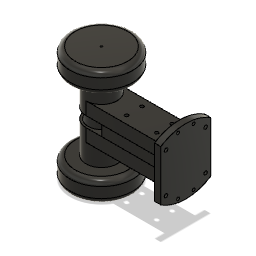
Supports projet fin de b3 (Autodesk Fusion 360 design; units mm, degrees)
Autodesk Fusion 360 part; units mm, degrees
note: some values were not read from the file. Set by a fixed rule: which sketch regions a step uses.
sketch "Esquisse1" plane through (0, 0, 0) normal (0, 1, 0) x (1, 0, 0)
  line L0 (0, 0) -> (0, 8.7) construction
  line L1 (0, -8.35) -> (1.45, -8.35)
  line L2 (0, 8.35) -> (1.45, 8.35)
  line L3 (0, -8.35) -> (-1.45, -8.35)
  circle A0 centre (0, 0) radius 2.9 construction
  circle A1 centre (0, 0) radius 9.45 construction
  line L4 (0, 0) -> (0, 1.3273)
  circle A2 centre (0, 0) radius 0.9
  line L5 (0, -8.7) -> (1.45, -8.7)
  line L6 (0, 8.35) -> (-1.45, 8.35)
  line L7 (0, 8.7) -> (-1.45, 8.7)
  line L8 (-6.6, 0) -> (-4.4, 0)
  circle A3 centre (5.5, 0.0034) radius 1.1
  line L9 (1.45, -8.7) -> (1.45, -8.35)
  line L10 (0, -8.7) -> (-1.45, -8.7)
  line L11 (1.45, 8.7) -> (1.45, 8.35)
  line L12 (-1.45, 8.7) -> (-1.45, 8.35)
  line L13 (0, 0) -> (-4.4, 0) construction
  circle A4 centre (-5.5, 0.0034) radius 1.1
  line L14 (0, 8.7) -> (1.45, 8.7)
  circle A5 centre (0, 0) radius 11.8 construction
  line L15 (0, 0) -> (0, 8.35) construction
  line L16 (-1.45, -8.7) -> (-1.45, -8.35)
  circle A6 centre (0, 0) radius 10.45
  circle A7 centre (0, 0) radius 12.8
  circle A8 centre (0, 0) radius 3.9
  circle A9 centre (0, 0) radius 14.8
  line L17 (0, 0) -> (-3.9, 0)
  line L18 (-3.9, 0) -> (-3.9, 3.9) construction
  line L19 (-3.9, 3.9) -> (0, 3.9) construction
  line L20 (0, 3.9) -> (0, 0)
  line L21 (0, 0) -> (-3.9, 3.9) construction
  circle A10 centre (-0.0034, 5.5) radius 1.1
  line L22 (-8.35, 0) -> (-8.35, 1.45)
  line L23 (-8.7, 0) -> (-8.7, -1.45)
  line L24 (-8.7, 1.45) -> (-8.35, 1.45)
  line L25 (-8.7, 0) -> (-8.7, 1.45)
  line L26 (-8.35, 0) -> (-8.35, -1.45)
  line L27 (-8.7, -1.45) -> (-8.35, -1.45)
  line L28 (8.7, 0) -> (8.7, 1.45)
  line L29 (8.35, 0) -> (8.35, -1.45)
  line L30 (8.7, 0) -> (8.7, -1.45)
  line L31 (8.7, 1.45) -> (8.35, 1.45)
  line L32 (8.35, 0) -> (8.35, 1.45)
  line L33 (8.7, -1.45) -> (8.35, -1.45)
  circle A11 centre (-0.0034, -5.5) radius 1.1
  circle A12 centre (0, 0) radius 30
  dimension "d1" = 5.8
  dimension "d2" = 18.9
  dimension "d3" = 23.6
  dimension "d5" = 2.2
  dimension "d7" = 8.7
  dimension "d8" = 8.35
  dimension "d9" = 1.45
  dimension "d10" = 1.45
  dimension "d11" = 1.8
  dimension "d12" = 1
  dimension "d13" = 1
  dimension "d14" = 1
  dimension "d15" = 3
  dimension "d157" = 5.4966
  dimension "d158" = 7.7829
  dimension "d159" = 5.5
  dimension "d171" = 60
  constraint coincident L0.start A0.centre
  constraint concentric A1 A5
  constraint horizontal L13
  constraint coincident L8.end A4
  constraint coincident L8.start A4
  constraint parallel L8 L13
  constraint perpendicular L4 L13
  constraint symmetric L4 A3 A4
  constraint perpendicular L0 L13
  constraint perpendicular L13 L15
  constraint perpendicular L6 L15
  constraint perpendicular L0 L7
  constraint symmetric L7.start L14.start L0
  constraint symmetric L2.start L6.start L0
  constraint symmetric L2.end L6.end L0
  constraint symmetric L11.start L7.end L0
  constraint symmetric L0.end L5.start L13
  constraint symmetric L2.start L1.start L13
  constraint symmetric L6.end L3.end L13
  constraint symmetric L10.end L7.end L13
  constraint symmetric L5.end L11.start L13
  constraint symmetric L1.start L2.start L13
  constraint symmetric L1.end L2.end L13
  constraint concentric A0 A2
  constraint perpendicular L17 L18
  constraint parallel L17 L19
  constraint parallel L18 L20
  constraint coincident A8 L17.end
  constraint coincident L13 L17.end
  constraint parallel L13 L17
  constraint symmetric L0.end L21 L23.start
  constraint symmetric L2.start L21 L22.start
  constraint symmetric L2.end L21 L26.end
  constraint symmetric L11.start L21 L23.end
  constraint symmetric L6.end L21 L22.end
  constraint symmetric L7.end L21 L24.start
  constraint symmetric A4 L21 A10
  constraint symmetric L10.end L21 L28.end
  constraint symmetric L5.end L21 L30.end
  constraint symmetric L1.start L21 L29.start
  constraint symmetric L1.end L21 L29.end
  constraint symmetric L5.start L21 L28.start
  constraint symmetric L3.end L21 L31.end
  constraint symmetric A3 L21 A11
  constraint concentric A1 A12
  measures "d1" diameter of A0
  measures "d2" diameter of A1
  measures "d3" diameter of A5
  measures "d5" diameter of A4
  measures "d7" distance of L0.start L0.end
  measures "d8" distance of L0.start L2.start
  measures "d9" distance of L0.end L7.end
  measures "d10" distance of L2.start L6.end
  measures "d11" diameter of A2
  measures "d157" horizontal distance of A4.centre A11.centre
  measures "d158" distance of A3.centre A11.centre
  measures "d159" horizontal distance of A4.centre L0.start
  measures "d171" diameter of A12
extrude "Extrusion1" add sketch "Esquisse1" along normal blind 30.1 contours A9 makes body 1
extrude "Extrusion2" add sketch "Esquisse1" along normal blind 2 contours L1 L3 L5 L9 L10 L16 | L2 L6 L7 L11 L12 L14 | A6 | A7 | L22 L23 L24 L25 L26 L27 | L28 L29 L30 L31 L32 L33 bodies 1
extrude "Extrusion16" add sketch "Esquisse1" against normal blind 20 separate body contours L1 L3 L5 L9 L10 L16 | L2 L6 L7 L11 L12 L14 | L4 A2 A8 L17 L20 | L4 A2 A8 L17 L20 | L8 A4 | L8 A4 | A3 | A6 | A7 | A9 | A10 | L22 L23 L24 L25 L26 L27 | L28 L29 L30 L31 L32 L33 | A11 | A12 makes body 2
fillet "Congé3" radius 5 2 edges at (-27.9698, -20, -10.8485) (-27.9698, 0, 10.8485) on bodies 2
ref_plane "Plan de construction1" through (0, 30.1, 0) normal (0, 1, 0) x (1, 0, 0)
sketch "Esquisse2" plane through (0, 30.1, 0) normal (0, 1, 0) x (1, 0, 0)
  circle A0 centre (0, 0) radius 14.8
  line L0 (0, 14.8) -> (15, 14.8)
  line L1 (15, 14.8) -> (15, -14.8) construction
  line L2 (0, -14.8) -> (15, -14.8)
  circle A1 centre (5.5, 0) radius 1
  circle A2 centre (-5.5, 0) radius 1
  line L3 (0, 0) -> (-2, 0)
  line L4 (0.0051, -2) -> (0, 0)
  line L5 (0, 0) -> (-2, -2) construction
  circle A3 centre (0, -5.5) radius 1
  circle A4 centre (0, 5.5) radius 1
  line L6 (0.0222, -8.6986) -> (1.4663, -8.6986)
  line L7 (1.4663, -8.6986) -> (1.4663, -8.3486)
  line L8 (1.4663, -8.3486) -> (0.0213, -8.3486)
  line L9 (0.0222, -8.6986) -> (-1.4219, -8.706)
  line L10 (-1.4237, -8.356) -> (0.0213, -8.3486)
  line L11 (-1.4219, -8.706) -> (-1.4237, -8.356)
  line L12 (0, 0) -> (-4.4, 0)
  line L13 (-1.4219, 8.706) -> (-1.4237, 8.356)
  line L14 (1.4663, 8.3486) -> (0.0213, 8.3486)
  line L15 (0.0222, 8.6986) -> (-1.4219, 8.706)
  line L16 (0.0222, 8.6986) -> (1.4663, 8.6986)
  line L17 (-1.4237, 8.356) -> (0.0213, 8.3486)
  line L18 (1.4663, 8.6986) -> (1.4663, 8.3486)
  line L19 (-8.356, -1.4237) -> (-8.3486, 0.0213)
  line L20 (-8.6986, 0.0222) -> (-8.6986, 1.4663)
  line L21 (-8.6986, 0.0222) -> (-8.706, -1.4219)
  line L22 (-8.3486, 1.4663) -> (-8.3486, 0.0213)
  line L23 (-8.706, -1.4219) -> (-8.356, -1.4237)
  line L24 (-8.6986, 1.4663) -> (-8.3486, 1.4663)
  line L25 (8.6986, 1.4663) -> (8.3486, 1.4663)
  line L26 (8.3486, 1.4663) -> (8.3486, 0.0213)
  line L27 (8.6986, 0.0222) -> (8.706, -1.4219)
  line L28 (8.356, -1.4237) -> (8.3486, 0.0213)
  line L29 (8.6986, 0.0222) -> (8.6986, 1.4663)
  line L30 (8.706, -1.4219) -> (8.356, -1.4237)
  line L31 (1.7678, 1.7678) -> (0, 0) construction
  line L32 (-10.4652, 10.4652) -> (0, 0) construction
  line L33 (11.8794, -9.051) -> (11.7834, -8.955)
  line L34 (-1.4106, 1.4178) -> (-1.4178, 1.4106)
  line L35 (-1.4106, -1.4178) -> (-1.4178, -1.4106)
  line L36 (-1.4142, -1.4142) -> (-1.407, -1.4214)
  line L37 (-1.4142, 1.4142) -> (-1.407, 1.4214)
  circle A5 centre (0, 0) radius 2.5
  line L38 (15, 14.8) -> (15, -14.8)
  line L39 (15, -14.8) -> (17, -14.8)
  line L40 (17, -14.8) -> (17, 14.8)
  line L41 (17, 14.8) -> (15, 14.8)
  line L42 (17, -14.8) -> (17, 14.8)
  line L43 (17, 14.8) -> (74.8, 14.8)
  line L44 (74.8, 14.8) -> (74.8, -14.8)
  line L45 (74.8, -14.8) -> (17, -14.8)
  line L46 (17, -14.8) -> (17, -17.3)
  line L47 (17, -17.3) -> (22, -17.3)
  line L48 (22, -14.8) -> (17, -14.8)
  line L49 (15, -14.8) -> (15, -19.3)
  line L50 (15, -19.3) -> (22, -19.3)
  line L51 (22, -19.3) -> (22, -17.3)
  line L52 (22, -14.8) -> (15, -14.8)
  line L53 (100.3975, 14.8) -> (100.3975, -14.8)
  line L54 (110.3975, -14.8) -> (110.3975, 14.8)
  line L55 (110.3975, 14.8) -> (100.3975, 14.8)
  line L56 (100.3975, -14.8) -> (110.3975, -14.8)
  line L57 (63.9025, 4.6) -> (76.9025, 4.6)
  line L58 (76.9025, 4.6) -> (76.9025, -4.6)
  line L59 (76.9025, -4.6) -> (63.9025, -4.6)
  line L60 (63.9025, -4.6) -> (63.9025, 4.6)
  line L61 (63.9025, 4.6) -> (76.9025, -4.6) construction
  line L62 (76.9025, 4.6) -> (63.9025, -4.6) construction
  line L63 (58.6988, -14.8) -> (58.6988, -31.5) construction
  line L64 (102.3975, -19.3) -> (95.3975, -19.3)
  line L65 (100.3975, -17.3) -> (95.3975, -17.3)
  line L66 (95.3975, -19.3) -> (95.3975, -17.3)
  line L67 (100.3975, -14.8) -> (100.3975, -17.3)
  line L68 (102.3975, -14.8) -> (102.3975, -19.3)
  line L69 (45.9, 14.8) -> (45.9, -14.8) construction
  line L70 (45.9, 0) -> (74.8, 14.8) construction
  line L71 (74.8, -14.8) -> (45.9, 0) construction
  line L72 (45.9, 0) -> (17, -14.8) construction
  line L73 (45.9, 0) -> (17, 14.8) construction
  circle A6 centre (31.45, 7.4) radius 1.6
  circle A7 centre (60.35, 7.4) radius 1.6
  circle A8 centre (31.45, -7.4) radius 1.6
  circle A9 centre (60.35, -7.4) radius 1.6
  line L74 (99.295, 0) -> (76.9025, 0) construction
  line L75 (100.3975, 0) -> (90.3975, 0) construction
  line L76 (90.3975, 0) -> (90.3975, 4.5)
  line L77 (90.3975, 4.5) -> (100.3975, 4.5)
  line L78 (100.3975, 4.5) -> (100.3975, 0)
  line L79 (90.3975, -4.5) -> (100.3975, -4.5)
  line L80 (90.3975, 0) -> (90.3975, -4.5)
  line L81 (74.8, -4.6) -> (74.8, 4.6)
  line L82 (63.9025, 0) -> (76.9025, 0)
  line L83 (90.3975, 0) -> (100.3975, 0)
  line L84 (22, 19.3) -> (22, 17.3)
  line L85 (17, 17.3) -> (22, 17.3)
  line L86 (17, 14.8) -> (17, 17.3)
  line L87 (15, 19.3) -> (22, 19.3)
  line L88 (15, 14.8) -> (15, 19.3)
  line L89 (45.9, 0) -> (85, 0) construction
  point P0 (70.4025, 0)
  dimension "d21" = 29.6
  dimension "d22" = 2
  dimension "d23" = 2
  dimension "d24" = 2
  dimension "d25" = 2
  dimension "d32" = 5
  dimension "d33" = 57.8
  dimension "d35" = 2
  dimension "d36" = 15
  dimension "d41" = 5.5
  dimension "d42" = 14.8
  dimension "d47" = 2.5
  dimension "d48" = 5
  dimension "d49" = 4.5
  dimension "d50" = 10
  dimension "d53" = 13
  dimension "d54" = 9.2
  dimension "d56" = 5
  dimension "d58" = 90
  dimension "d59" = 5
  dimension "d60" = 29.6
  dimension "d61" = 3.2
  dimension "d62" = 3.2
  dimension "d63" = 3.2
  dimension "d64" = 3.2
  dimension "d66" = 25.5975
  dimension "d70" = 46.9025
  dimension "d72" = 10
  dimension "d73" = 4.5
  constraint coincident A0.centre L3.start
  constraint coincident A0 L0.start
  constraint tangent A0 L0
  constraint horizontal L0
  constraint perpendicular L0 L1
  constraint coincident A0 L2.start
  constraint tangent A0 L2
  constraint perpendicular L1 L2
  constraint horizontal L3
  constraint symmetric A2 L5 A3
  constraint symmetric A1 L5 A4
  constraint horizontal L6
  constraint perpendicular L6 L7
  constraint perpendicular L7 L8
  constraint symmetric L4 L6.start L9.start
  constraint symmetric L4 L6.end L9.end
  constraint symmetric L4 L7.end L10.start
  constraint symmetric L4 L8.end L10.end
  constraint symmetric L6.start L12 L15.start
  constraint symmetric L6.end L12 L16.end
  constraint symmetric L7.end L12 L14.start
  constraint symmetric L8.end L12 L14.end
  constraint symmetric L9.end L12 L13.start
  constraint symmetric L10.start L12 L13.end
  constraint symmetric L5 L6.start L20.start
  constraint symmetric L5 L6.end L20.end
  constraint symmetric L5 L7.end L22.start
  constraint symmetric L5 L8.end L19.end
  constraint symmetric L5 L9.end L21.end
  constraint symmetric L5 L10.start L19.start
  constraint symmetric L5 L14.end L26.end
  constraint symmetric L5 L13.start L27.end
  constraint symmetric L5 L13.end L28.start
  constraint symmetric L5 L14.start L25.end
  constraint symmetric L5 L16.end L25.start
  constraint symmetric L5 L15.start L27.start
  constraint symmetric L4 A0.centre L3.start
  constraint symmetric L12 L34.end L35.end
  constraint symmetric L12 L36.end L37.end
  constraint coincident A0 L32.start
  constraint coincident L5 L36.start
  constraint coincident L32 L37.start
  constraint perpendicular L38 L39
  constraint parallel L38 L40
  constraint parallel L39 L41
  constraint perpendicular L42 L43
  constraint parallel L42 L44
  constraint parallel L43 L45
  constraint coincident A5 L31.start
  constraint coincident A0 L33.end
  constraint perpendicular L46 L47
  constraint parallel L47 L48
  constraint perpendicular L39 L46
  constraint perpendicular L49 L50
  constraint parallel L49 L51
  constraint parallel L50 L52
  constraint perpendicular L47 L49
  constraint parallel L53 L54
  constraint perpendicular L43 L53
  constraint perpendicular L54 L56
  constraint horizontal L57
  constraint perpendicular L57 L58
  constraint parallel L57 L59
  constraint parallel L58 L60
  constraint coincident L61 P0
  constraint coincident L62 P0
  constraint symmetric L1.end L63 L68.start
  constraint symmetric L39.end L63 L53.end
  constraint symmetric L46.end L63 L65.start
  constraint symmetric L47.end L63 L65.end
  constraint symmetric L49.end L63 L64.start
  constraint symmetric L50.end L63 L64.end
  constraint coincident L45 L63.start
  constraint midpoint L43 L69.start
  constraint midpoint L45 L69.end
  constraint midpoint L69 L70.start
  constraint midpoint L73 A6.centre
  constraint midpoint L70 A7.centre
  constraint midpoint L72 A8.centre
  constraint midpoint L71 A9.centre
  constraint perpendicular L58 L74
  constraint coincident L58 L74.end
  constraint perpendicular L75 L76
  constraint parallel L75 L77
  constraint parallel L76 L78
  constraint perpendicular L53 L75
  constraint midpoint L53 L75.start
  constraint symmetric L76.start L75 L80.start
  constraint symmetric L76.end L75 L79.start
  constraint symmetric L77.end L75 L79.end
  constraint coincident L59 L81.start
  constraint coincident L44 L81.start
  constraint coincident L57 L81.end
  constraint coincident L44 L81.end
  constraint midpoint L60 L82.start
  constraint perpendicular L58 L82
  constraint symmetric L39.end L74 L40.end
  constraint symmetric L46.end L74 L85.start
  constraint symmetric L47.end L74 L84.end
  constraint symmetric L49.end L74 L87.start
  constraint symmetric L50.end L74 L84.start
  constraint symmetric L1.end L74 L0.end
  constraint perpendicular L69 L89
  constraint collinear L82 L89
  measures "d21" diameter of A0
  measures "d22" diameter of A1
  measures "d23" diameter of A2
  measures "d24" distance of A0.centre L3.end
  measures "d25" distance of A0.centre L4.start
  measures "d32" diameter of A5
  measures "d33" distance of L39.end L44.end
  measures "d35" distance of L38 L42
  measures "d36" distance of L0.start L0.end
  measures "d41" distance of A0.centre A1.centre
  measures "d42" distance of L0 A1.centre
  measures "d47" distance of L39.end L46.end
  measures "d48" distance of L39.end L48.start
  measures "d49" distance of L1.end L49.end
  measures "d50" distance of L53 L54
  measures "d53" distance of L58.end L59.end
  measures "d54" distance of L57.end L58.end
  measures "d56" distance of L65.start L65.end
  measures "d58" angle of L56 L68
  measures "d59" distance of L53 L66
  measures "d60" distance of L55 L56
  measures "d61" diameter of A6
  measures "d62" diameter of A7
  measures "d63" diameter of A8
  measures "d64" diameter of A9
  measures "d66" distance of L44 L53
  measures "d70" distance of L40 L60
  measures "d72" distance of L75.start L75.end
  measures "d73" distance of L75.start L77.end
extrude "Extrusion4" add sketch "Esquisse2" against normal blind 12.25 contours A0 L0 L2 L38 | L38 L39 L40 L41 L42 L52 | L40 L42 L43 L44 L45 L48 L52 L57 L59 L60 | L44 L57 L60 L81 L82 | L44 L59 L60 L81 L82 bodies 1
extrude "Extrusion9" add sketch "Esquisse2" against normal blind 6.24 contours L40 L42 L43 L44 L45 L48 L52 L57 L59 L60 | L44 L57 L60 L81 L82 | L44 L59 L60 L81 L82 bodies 1
extrude "Extrusion5" add sketch "Esquisse2" along normal blind -12.25 and the other way blind -12.25 separate body contours L53 L54 L55 L56 L78 makes body 3
revolve "Révolution2" add sketch "Esquisse2" angle 360 about axis through (99.295, 30.1, 0) along (-1, 0, 0) contours L53 L76 L77 L78 L83 bodies 3
sketch "Esquisse3" plane through (110.3975, 0, 0) normal (1, 0, 0) x (0, 0, -1)
  circle A0 centre (18.95, 48.95) radius 1.65
  circle A1 centre (18.95, 11.05) radius 1.65
  circle A2 centre (-18.95, 11.05) radius 1.65
  line L0 (-18.95, 48.95) -> (18.95, 11.05) construction
  line L1 (18.95, 48.95) -> (-18.95, 11.05) construction
  circle A3 centre (-18.95, 48.95) radius 1.65
  line L2 (-24, 6) -> (-24, 54.35)
  line L3 (24, 54.35) -> (24, 6)
  line L4 (24, 6) -> (-24, 54.35) construction
  line L5 (-24, 6) -> (24, 54.35) construction
  circle A4 centre (-7.5, 57.55) radius 1.4
  circle A5 centre (7.5, 57.55) radius 1.4
  line L6 (24, 30.175) -> (39, 30.175)
  circle A6 centre (-7.5, 2.8) radius 1.4
  circle A7 centre (7.5, 2.8) radius 1.4
  arc A8 (-24, 6) -> (24, 6) centre (0, 42.9444) ccw
  arc A9 (24, 54.35) -> (-24, 54.35) centre (0, 17.4056) ccw
  point P0 (0, 9)
  point P1 (0, 30.175)
  point P2 (0, 30.175)
  dimension "d132" = 3.3
  constraint coincident A0.centre L1.start
  constraint coincident A2.centre L1.end
  constraint coincident L0.start A3.centre
  constraint coincident A1.centre L0.end
  constraint perpendicular L0 L1
  constraint parallel L2 L3
  constraint coincident L4 P2
  constraint coincident L5 P2
  constraint coincident P2 P1
  constraint midpoint L3 L6.start
  constraint perpendicular L3 L6
  constraint symmetric A4 L6 A6
  constraint symmetric A5 L6 A7
  constraint symmetric L3.end L6 L3.start
  constraint symmetric L2.start L6 L2.end
  constraint symmetric L6 A8 A9
  measures "d132" diameter of A3
extrude "Extrusion8" add sketch "Esquisse2" along normal blind 10 separate body contours L38 L39 L40 L41 L42 L52 | L40 L42 L43 L44 L45 L48 L52 L57 L59 L60 | L44 L57 L60 L81 L82 | L44 L59 L60 L81 L82 makes body 4
copy_body "Copier/Coller des corps3" bodies 1 makes body 5
move_body "Déplacer5" bodies 5 to x (1, 0, 0) y (0, -1, 0) z (0, 0, -1) at (0, 90, 0.4)
move_body "Déplacer10" bodies 5 to x (1, 0, 0) y (0, 1, 0) z (0, 0, 1) at (0, -19.8, -0.4)
ref_plane "Plan de construction2" through (44.9, 35.1, 0) normal (0, -1, 0) x (-1, 0, 0)
sketch "Esquisse5" plane through (74.8, 0, 0) normal (1, 0, 0) x (0, 0, -1)
  line L0 (-14.8, 30.1) -> (14.8, 30.1)
  line L1 (14.8, 30.1) -> (14.8, 40.1)
  line L2 (14.8, 40.1) -> (-14.8, 40.1)
  line L3 (-14.8, 40.1) -> (-14.8, 30.1)
  line L4 (0, 40.1) -> (0, 26) construction
  line L5 (0, 40.1) -> (26, 40.1) construction
  circle A0 centre (0, 35.1) radius 4.6
  point P0 (0, 40.1)
  dimension "d151" = 9.2
  dimension "d152" = 5
  constraint midpoint L2 P0
  constraint coincident P0 L4.start
  constraint perpendicular L2 L4
  constraint perpendicular L4 L5
  constraint coincident L4 A0.centre
  measures "d151" diameter of A0
  measures "d152" distance of L5 A0.centre
extrude "Extrusion14" cut sketch "Esquisse5" against normal blind 9.2 contours A0 bodies 4
extrude "Extrusion11" add sketch "Esquisse3" against normal blind 10 bodies 3
extrude "Extrusion12" cut sketch "Esquisse3" against normal blind 4 contours A0 | A1 | A2 | A3 | L2 L3 A8 A9 bodies 3
move_body "Déplacer7" bodies 3 to x (1, 0, 0) y (0, 1, 0) z (0, 0, 1) at (4, 0, 0)
sketch "Esquisse6" plane through (0, 0, -14.8) normal (0, 0, -1) x (-1, 0, 0)
  line L0 (-74.8, 30.1) -> (-15, 30.1)
  line L1 (-15, 30.1) -> (-15, 40.1)
  line L2 (-15, 40.1) -> (-74.8, 40.1)
  line L3 (-74.8, 40.1) -> (-74.8, 30.1)
  line L4 (-67.35, 45.75) -> (-67.35, 48.35) construction
  line L5 (-67.35, 48.35) -> (-64.75, 48.35) construction
  line L6 (-64.75, 45.75) -> (-67.35, 45.75) construction
  line L7 (-64.75, 48.35) -> (-64.75, 45.75) construction
  line L8 (-66.05, 47.05) -> (-14.95, 22.95) construction
  line L9 (-14.95, 22.95) -> (-14.95, 47.05) construction
  line L10 (-14.95, 47.05) -> (-66.05, 22.95) construction
  line L11 (-66.05, 22.95) -> (-66.05, 47.05) construction
  line L12 (-14.95, 47.05) -> (-66.05, 47.05) construction
  line L13 (-40.5, 40.1) -> (-40.5, 35) construction
  circle A0 centre (-66.05, 47.05) radius 2.3
  circle A1 centre (-14.95, 47.05) radius 2.3
  circle A2 centre (-14.95, 22.95) radius 2.3
  circle A3 centre (-66.05, 22.95) radius 2.3
  point P0 (-40.5, 40.1)
  dimension "d155" = 2.6
  dimension "d156" = 2.6
  dimension "d161" = 56.498
  dimension "d162" = 51.1
  dimension "d163" = 24.1
  dimension "d165" = 4.6
  dimension "d166" = 4.6
  dimension "d167" = 4.6
  dimension "d168" = 4.6
  constraint horizontal L5
  constraint horizontal L6
  constraint vertical L4
  constraint vertical L9
  constraint perpendicular L6 L11
  constraint perpendicular L11 L12
  constraint midpoint L10 L13.end
  constraint coincident L2 P0
  constraint coincident P0 L13.start
  measures "d155" distance of L4.end L5.end
  measures "d156" distance of L4.start L4.end
  measures "d161" distance of L8.start L8.end
  measures "d162" horizontal distance of L9.end L10.end
  measures "d163" distance of L10.end L8.start
  measures "d165" diameter of A0
  measures "d166" diameter of A1
  measures "d167" diameter of A2
  measures "d168" diameter of A3
extrude "Extrusion15" cut sketch "Esquisse6" against normal blind 4 contours A0 | A1 | A2 | A3 bodies 1 5
copy_body "Corps->Comp1" bodies 3 removing the originals makes body 6 in component "support haut"
copy_body "Corps->Comp2" bodies 1 removing the originals makes body 7 in component "support moteur "
copy_body "Corps->Comp3" bodies 5 removing the originals makes body 8 in component "support moteur  2"
copy_body "Corps->Comp4" bodies 4 removing the originals makes body 9 in component "paroie centrale"
move_body "Déplacer2" bodies 6 to x (1, 0, 0) y (0, 1, 0) z (0, 0, 1) at (-29.5975, 5, 0) in component "support haut"
copy_body "Copier/Coller des corps4" bodies 2 makes body 10
move_body "Déplacer11" bodies 10 to x (1, 0, 0) y (0, 1, 0) z (0, 0, 1) at (0, 90.2, 0)
copy_body "Corps->Comp5" bodies 2 removing the originals makes body 11 in component "roue1"
copy_body "Corps->Comp6" bodies 10 removing the originals makes body 12 in component "roue2"
component "support haut" placed x (1, 0, 0) y (0, 1, 0) z (0, 0, 1) at (0, 0, 0)
component "support moteur " placed x (1, 0, 0) y (0, 1, 0) z (0, 0, 1) at (0, 0, 0)
component "support moteur  2" placed x (1, 0, 0) y (0, 1, 0) z (0, 0, 1) at (0, 0, 0)
component "paroie centrale" placed x (1, 0, 0) y (0, 1, 0) z (0, 0, 1) at (0, 0, 0)
component "roue1" placed x (1, 0, 0) y (0, 1, 0) z (0, 0, 1) at (0, 0, 0)
component "roue2" placed x (1, 0, 0) y (0, 1, 0) z (0, 0, 1) at (0, 0, 0)
equation "d16 = 27.1 mm + 1 mm + 2 mm"
equation "d33 = 55.8 mm + 2 mm"
equation "d53 = 11 mm + 2 mm"
equation "d73 = 5.000 mm - 0.5 mm"
equation "d74 = ( -22.50 / 2 ) * 1 mm - 1 mm"
equation "d78 = ( -22.50 / 2 ) * 1 mm - 1 mm"
equation "d80 = ( -22.50 / 2 ) * 1 mm - 1 mm"
equation "d96 = -12.25 mm + 6.01 mm"
equation "d165 = 2.60 mm + 2 mm"
equation "d166 = 2.60 mm + 2 mm"
equation "d167 = 2.60 mm + 2 mm"
equation "d168 = 2.60 mm + 2 mm"
named bodies: "support moteur", "support haut", "paroie centrale", "support moteur  2", "roue1", "roue2"
